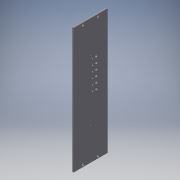
# Autodesk Inventor part: Large_frontplatte
Saved by Autodesk Inventor 2018 (Build 220112000, 112)
## iProperties
Created: 2018-06-01
Part Number: Large_frontplatte
Material: Generic
Document SubType Name: Modeling
Designer: David
Density: 1 g/cm^3
Appearance: Default
Author: David
Autodesk Inventor part; units mm, degrees
ref_plane "YZ Plane" through (0, 0, 0) normal (1, 0, 0) x (0, 1, 0)
ref_plane "XZ Plane" through (0, 0, 0) normal (0, 1, 0) x (-1, 0, 0)
ref_plane "XY Plane" through (0, 0, 0) normal (0, 0, 1) x (1, 0, 0)
sketch "Sketch1" plane through (0, 0, 0) normal (1, 0, 0) x (0, 1, 0)
  line L0 (-66, -242.5) -> (66, -242.5)
  line L1 (66, -242.5) -> (66, 242.5)
  line L2 (66, 242.5) -> (-66, 242.5)
  line L3 (-66, 242.5) -> (-66, -242.5)
  line L4 (-66, -242.5) -> (66, 242.5) construction
  line L5 (66, -242.5) -> (-66, 242.5) construction
  point P0 (0, 0)
  dimension "d0" = 132
  dimension "d1" = 485
  constraints: 12 end point, 2 midpoint, 2 parallel, 1 horizontal, 1 perpendicular
  measures "d0" distance of L2.end L1.end
  measures "d1" distance of L1.end L0.end
extrude "Extrusion1" add sketch "Sketch1" along normal blind 5
sketch "Sketch2" plane through (5, 0, 0) normal (1, 0, 0) x (0, 0, -1)
  line L0 (-242.5, -66) -> (242.5, -66) projected
  line L1 (-242.5, 66) -> (-242.5, -66) projected
  line L2 (0, 66) -> (0, -66) construction
  line L3 (-242.5, 0) -> (242.5, 0) construction
  line L4 (-230.4092, -32.335) -> (-238.2708, -32.335)
  line L5 (-238.2708, -25.405) -> (-230.4092, -25.405)
  line L6 (-230.4092, -32.335) -> (-238.2708, -25.405) construction
  line L7 (-238.2708, -32.335) -> (-230.4092, -25.405) construction
  arc A0 (-238.2708, -25.405) -> (-238.2708, -32.335) centre (-234.34, -28.87) ccw
  arc A1 (-230.4092, -32.335) -> (-230.4092, -25.405) centre (-234.34, -28.87) ccw
  line L8 (238.2708, -32.335) -> (230.4092, -32.335)
  line L9 (230.4092, -25.405) -> (238.2708, -25.405)
  line L10 (238.2708, -32.335) -> (230.4092, -25.405) construction
  line L11 (230.4092, -32.335) -> (238.2708, -25.405) construction
  arc A2 (230.4092, -25.405) -> (230.4092, -32.335) centre (234.34, -28.87) ccw
  arc A3 (238.2708, -32.335) -> (238.2708, -25.405) centre (234.34, -28.87) ccw
  line L12 (-230.4092, 25.405) -> (-238.2708, 25.405)
  line L13 (-238.2708, 32.335) -> (-230.4092, 32.335)
  line L14 (-230.4092, 25.405) -> (-238.2708, 32.335) construction
  line L15 (-238.2708, 25.405) -> (-230.4092, 32.335) construction
  arc A4 (-238.2708, 32.335) -> (-238.2708, 25.405) centre (-234.34, 28.87) ccw
  arc A5 (-230.4092, 25.405) -> (-230.4092, 32.335) centre (-234.34, 28.87) ccw
  line L16 (238.2708, 25.405) -> (230.4092, 25.405)
  line L17 (230.4092, 32.335) -> (238.2708, 32.335)
  line L18 (238.2708, 25.405) -> (230.4092, 32.335) construction
  line L19 (230.4092, 25.405) -> (238.2708, 32.335) construction
  arc A6 (230.4092, 32.335) -> (230.4092, 25.405) centre (234.34, 28.87) ccw
  arc A7 (238.2708, 25.405) -> (238.2708, 32.335) centre (234.34, 28.87) ccw
  line L20 (121, -42.5) -> (-121, -42.5)
  line L21 (-121, -42.5) -> (-121, 42.5)
  line L22 (-121, 42.5) -> (121, 42.5)
  line L23 (121, 42.5) -> (121, -42.5)
  line L24 (121, -42.5) -> (-121, 42.5) construction
  line L25 (-121, -42.5) -> (121, 42.5) construction
  circle A8 centre (-117.9, 0) radius 1.65
  line L26 (-6.7, 0) -> (478.3, 0) construction
  circle A9 centre (117.9, 0) radius 1.65
  circle A10 centre (-103, 7.5) radius 2.5
  line L27 (-106.55, 20.5506) -> (-106.55, 24.4494)
  line L28 (-99.45, 24.4494) -> (-99.45, 20.5506)
  line L29 (-99.45, 20.5506) -> (-106.55, 24.4494) construction
  line L30 (-106.55, 20.5506) -> (-99.45, 24.4494) construction
  arc A11 (-106.55, 20.5506) -> (-99.45, 20.5506) centre (-103, 22.5) ccw
  arc A12 (-99.45, 24.4494) -> (-106.55, 24.4494) centre (-103, 22.5) ccw
  line L31 (-220.5, 0) -> (264.5, 0) construction
  line L32 (143, -42.5) -> (-99, 42.5) construction
  circle A13 centre (-81, 7.5) radius 2.5
  arc A14 (-77.45, 24.4494) -> (-84.55, 24.4494) centre (-81, 22.5) ccw
  arc A15 (-84.55, 20.5506) -> (-77.45, 20.5506) centre (-81, 22.5) ccw
  line L33 (-84.55, 20.5506) -> (-84.55, 24.4494)
  line L34 (-77.45, 24.4494) -> (-77.45, 20.5506)
  line L35 (-84.55, 20.5506) -> (-77.45, 24.4494) construction
  line L36 (-77.45, 20.5506) -> (-84.55, 24.4494) construction
  line L37 (-198.5, 0) -> (286.5, 0) construction
  line L38 (165, -42.5) -> (-77, 42.5) construction
  circle A16 centre (-59, 7.5) radius 2.5
  arc A17 (-55.45, 24.4494) -> (-62.55, 24.4494) centre (-59, 22.5) ccw
  arc A18 (-62.55, 20.5506) -> (-55.45, 20.5506) centre (-59, 22.5) ccw
  line L39 (-62.55, 20.5506) -> (-62.55, 24.4494)
  line L40 (-55.45, 24.4494) -> (-55.45, 20.5506)
  line L41 (-62.55, 20.5506) -> (-55.45, 24.4494) construction
  line L42 (-55.45, 20.5506) -> (-62.55, 24.4494) construction
  line L43 (-176.5, 0) -> (308.5, 0) construction
  line L44 (187, -42.5) -> (-55, 42.5) construction
  circle A19 centre (-37, 7.5) radius 2.5
  arc A20 (-33.45, 24.4494) -> (-40.55, 24.4494) centre (-37, 22.5) ccw
  arc A21 (-40.55, 20.5506) -> (-33.45, 20.5506) centre (-37, 22.5) ccw
  line L45 (-40.55, 20.5506) -> (-40.55, 24.4494)
  line L46 (-33.45, 24.4494) -> (-33.45, 20.5506)
  line L47 (-40.55, 20.5506) -> (-33.45, 24.4494) construction
  line L48 (-33.45, 20.5506) -> (-40.55, 24.4494) construction
  line L49 (-154.5, 0) -> (330.5, 0) construction
  line L50 (209, -42.5) -> (-33, 42.5) construction
  circle A22 centre (-15, 7.5) radius 2.5
  arc A23 (-11.45, 24.4494) -> (-18.55, 24.4494) centre (-15, 22.5) ccw
  arc A24 (-18.55, 20.5506) -> (-11.45, 20.5506) centre (-15, 22.5) ccw
  line L51 (-18.55, 20.5506) -> (-18.55, 24.4494)
  line L52 (-11.45, 24.4494) -> (-11.45, 20.5506)
  line L53 (-18.55, 20.5506) -> (-11.45, 24.4494) construction
  line L54 (-11.45, 20.5506) -> (-18.55, 24.4494) construction
  line L55 (-132.5, 0) -> (352.5, 0) construction
  line L56 (231, -42.5) -> (-11, 42.5) construction
  circle A25 centre (7, 7.5) radius 2.5
  arc A26 (10.55, 24.4494) -> (3.45, 24.4494) centre (7, 22.5) ccw
  arc A27 (3.45, 20.5506) -> (10.55, 20.5506) centre (7, 22.5) ccw
  line L57 (3.45, 20.5506) -> (3.45, 24.4494)
  line L58 (10.55, 24.4494) -> (10.55, 20.5506)
  line L59 (3.45, 20.5506) -> (10.55, 24.4494) construction
  line L60 (10.55, 20.5506) -> (3.45, 24.4494) construction
  arc A28 (-121, 42.5) -> (-121, -42.5) centre (329.563, 0) ccw
  arc A29 (121, -42.5) -> (121, 42.5) centre (-329.563, 0) ccw
  line L61 (93.5, 43.5) -> (-93.5, 43.5)
  line L62 (-93.5, 43.5) -> (-93.5, 58.58)
  line L63 (-93.5, 58.58) -> (93.5, 58.58)
  line L64 (93.5, 58.58) -> (93.5, 43.5)
  line L65 (93.5, 43.5) -> (-93.5, 58.58) construction
  line L66 (-93.5, 43.5) -> (93.5, 58.58) construction
  line L67 (242.5, 66) -> (-242.5, 66) projected
  circle A30 centre (93.5, 51.5) radius 2.1
  circle A31 centre (-93.5, 51.5) radius 2.1
  line L68 (93.5, -58.58) -> (-93.5, -58.58)
  line L69 (-93.5, -58.58) -> (-93.5, -43.5)
  line L70 (-93.5, -43.5) -> (93.5, -43.5)
  line L71 (93.5, -43.5) -> (93.5, -58.58)
  line L72 (93.5, -58.58) -> (-93.5, -43.5) construction
  line L73 (-93.5, -58.58) -> (93.5, -43.5) construction
  circle A32 centre (93.5, -51.5) radius 2.1
  circle A33 centre (-93.5, -51.5) radius 2.1
  point P0 (0, 0)
  point P1 (-103, 22.5)
  point P2 (-81, 22.5)
  point P3 (-59, 22.5)
  point P4 (-37, 22.5)
  point P5 (-15, 22.5)
  point P6 (7, 22.5)
  point P7 (0, 51.04)
  point P8 (0, -51.04)
  dimension "d7" = 28.87
  dimension "d10" = 234.34
  dimension "d11" = 5.24
  dimension "d12" = 6.93
  dimension "d15" = 468.68
  dimension "d18" = 57.74
  dimension "d21" = 242
  dimension "d22" = 85
  dimension "d23" = 117.9
  dimension "d24" = 42.5
  dimension "d25" = 3.3
  dimension "d28" = 235.8
  dimension "d33" = 117.9
  dimension "d35" = 5
  dimension "d37" = 20
  dimension "d38" = 18
  dimension "d39" = 15
  dimension "d40" = 4.05
  dimension "d41" = 7.1
  dimension "d44" = 22
  dimension "d51" = 452.563
  dimension "d52" = 452.563
  dimension "d53" = 7.42
  dimension "d54" = 15.08
  dimension "d55" = 187
  dimension "d56" = 4.2
  dimension "d57" = 8
  dimension "d58" = 4.2
  dimension "d59" = 8
  dimension "d72" = 15.08
  dimension "d73" = 187
  dimension "d74" = 4.2
  dimension "d76" = 4.2
  dimension "d78" = 7.42
  dimension "d79" = 8
  dimension "d80" = 8
  constraints: 142 end point, 44 point on circle, 34 centre point, 29 midpoint, 9 parallel, 8 horizontal, 5 point on line, 3 perpendicular, 1 vertical, 1 vertical alignment, 138 other
  measures "d7" distance from line of L3 A0.centre
  measures "d10" distance from line of A0.centre L2
  measures "d11" radius of A0
  measures "d12" distance between parallel lines of L4 L5
  measures "d15" distance of A0.centre A2.centre
  measures "d18" distance of A0.centre A4.centre
  measures "d21" distance of L21.end L22.end
  measures "d22" distance of L20.end L21.end
  measures "d23" distance from line of L2 A8.centre
  measures "d24" distance from line of L20 A8.centre
  measures "d25" diameter of A8
  measures "d28" distance of L3.start L26.start
  measures "d33" distance from line of L2 A9.centre
  measures "d35" diameter of A10
  measures "d37" distance from line of L22 A11.centre
  measures "d38" distance from line of L21 A11.centre
  measures "d39" distance of A10.centre A11.centre
  measures "d40" radius of A12
  measures "d41" distance between parallel lines of L28 L27
  measures "d44" distance of L3.start L31.start
  measures "d51" radius of A28
  measures "d52" radius of A29
  measures "d53" distance between parallel lines of L67 L63
  measures "d54" distance of L61.end L62.end
  measures "d55" distance of L62.end L63.end
  measures "d56" diameter of A30
  measures "d57" distance from line of L61 A30.centre
  measures "d58" diameter of A31
  measures "d59" distance from line of A31.centre L61
  measures "d72" distance of L68.end L70.start
  measures "d73" distance of L70.start L71.start
  measures "d74" diameter of A32
  measures "d76" diameter of A33
  measures "d78" distance between parallel lines of L0 L68
  measures "d79" distance from line of L70 A33.centre
  measures "d80" distance from line of L70 A32.centre
extrude "Extrusion2" cut sketch "Sketch2" against normal blind 5 contours L4 A0 L5 A1 | L8 A2 L9 A3 | L12 A4 L13 A5 | L16 A6 L17 A7 | A8 | A9 | A10 | L27 A12 L28 A11 | A13 | L34 A15 L33 A14 | A16 | L40 A18 L39 A17 | A19 | L46 A21 L45 A20 | A22 | L52 A24 L51 A23 | A25 | L58 A27 L57 A26 | A30 L64 | L64 A30 | A31 L62 | L62 A31 | A32 L71 | L71 A32 | A33 L69 | L69 A33
body "Solid1"
